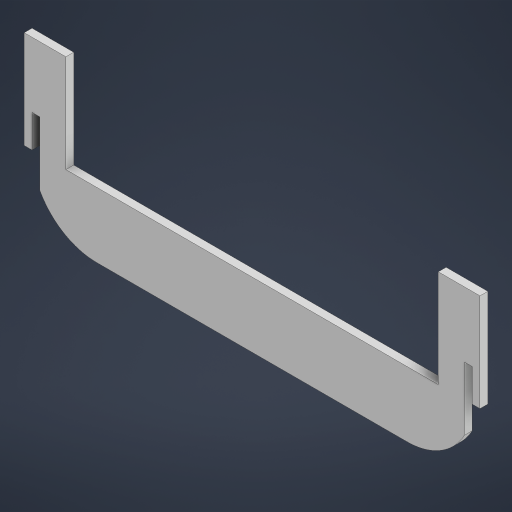
# Autodesk Inventor part: Battery_container_main
Saved by Autodesk Inventor 2024 (Build 280153000, 153)
## iProperties
Created: 2024-02-27
Part Number: Battery_container_main
Material: Generic
Document SubType Name: Modeling
Designer: calvi
Density: 1 g/cm^3
Appearance: Default
Author: calvi
Autodesk Inventor part; units mm, degrees
ref_plane "YZ Plane" through (0, 0, 0) normal (1, 0, 0) x (0, 1, 0)
ref_plane "XZ Plane" through (0, 0, 0) normal (0, 1, 0) x (-1, 0, 0)
ref_plane "XY Plane" through (0, 0, 0) normal (0, 0, 1) x (1, 0, 0)
sketch "Sketch1" plane through (0, 0, 0) normal (0, 0, 1) x (1, 0, 0)
  line L0 (0, 0) -> (171.704, 0)
  line L1 (171.704, 0) -> (171.704, 63.5)
  line L2 (171.704, 63.5) -> (0, 63.5)
  line L3 (0, 63.5) -> (0, 0)
  arc A0 (0, 25.4) -> (25.4, 0) centre (25.4, 25.4) ccw
  arc A1 (146.304, 0) -> (171.704, 25.4) centre (146.304, 25.4) ccw
  dimension "d0" = 171.704
  dimension "d1" = 63.5
  dimension "d2" = 50.8
  dimension "d3" = 50.8
  constraints: 8 end point, 4 point on circle, 4 point on line, 4 tangent, 2 centre point, 2 parallel, 1 horizontal, 1 perpendicular
  measures "d0" distance of L2.end L1.end
  measures "d1" distance of L1.end L0.end
  measures "d2" diameter of A0
  measures "d3" diameter of A1
extrude "Extrusion1" add sketch "Sketch1" along normal blind 3.048 contours A0 L3 L2 L1 A1 L0
sketch "Sketch3" plane through (0, 25.4, 0) normal (-1, 0, 0) x (0, 0, 1)
  line L0 (0, 38.1) -> (0, 0) projected
  line L1 (3.048, -25.4) -> (3.048, 0) projected
  line L2 (0, 38.1) -> (3.048, 38.1)
  line L3 (3.048, 38.1) -> (3.048, 0)
  line L4 (3.048, 0) -> (0, 0)
  line L5 (0, 0) -> (0, 38.1)
  point P0 (0, -25.4)
  constraints: 8 end point, 2 parallel, 1 horizontal, 1 perpendicular
extrude "Extrusion3" add sketch "Sketch3" along normal blind 3.048
sketch "Sketch4" plane through (171.704, 25.4, 0) normal (1, 0, 0) x (0, 0, -1)
  line L0 (-3.048, 38.1) -> (0, 38.1) projected
  line L1 (0, 0) -> (0, -25.4) projected
  line L2 (-3.048, 38.1) -> (0, 38.1)
  line L3 (0, 38.1) -> (0, 0)
  line L4 (0, 0) -> (-3.048, 0)
  line L5 (-3.048, 0) -> (-3.048, 38.1)
  point P0 (0, -25.4)
  constraints: 8 end point, 2 parallel, 1 horizontal, 1 perpendicular
extrude "Extrusion4" add sketch "Sketch4" along normal blind 3.048
sketch "Sketch5" plane through (0, 0, 3.048) normal (0, 0, 1) x (1, 0, 0)
  line L0 (0, 0) -> (3.048, 0)
  line L1 (3.048, 0) -> (3.048, 38.1)
  line L2 (3.048, 38.1) -> (0, 38.1)
  line L3 (0, 38.1) -> (0, 0)
  line L4 (-3.048, 63.5) -> (174.752, 63.5) projected
  line L5 (85.852, 63.5) -> (85.852, 0)
  line L6 (25.4, 0) -> (146.304, 0) projected
  line L7 (171.704, 0) -> (168.656, 0)
  line L8 (168.656, 0) -> (168.656, 38.1)
  line L9 (168.656, 38.1) -> (171.704, 38.1)
  line L10 (171.704, 38.1) -> (171.704, 0)
  point P0 (1.524, 0)
  point P1 (170.18, 0)
  dimension "d17" = 38.1
  dimension "d18" = 3.048
  constraints: 18 end point, 5 symmetric about line, 3 midpoint, 2 parallel, 1 horizontal, 1 perpendicular
  measures "d17" distance from line of L2 point (1.524, 0)
  measures "d18" distance between parallel lines of L3 L1
extrude "Extrusion5" cut sketch "Sketch5" against normal through all
sketch "Sketch6" plane through (0, 0, 3.048) normal (0, 0, 1) x (1, 0, 0)
  line L0 (-3.048, 63.5) -> (174.752, 63.5) projected
  line L1 (13.208, 63.5) -> (158.496, 63.5)
  line L2 (158.496, 63.5) -> (158.496, 25.4)
  line L3 (158.496, 25.4) -> (13.208, 25.4)
  line L4 (13.208, 25.4) -> (13.208, 63.5)
  line L5 (3.048, 38.1) -> (3.048, 13.3357) projected
  line L6 (168.656, 13.3357) -> (168.656, 38.1) projected
  line L7 (25.4, 0) -> (146.304, 0) projected
  point P0 (0, 0)
  point P1 (158.496, 63.5)
  dimension "d21" = 10.16
  dimension "d22" = 10.16
  dimension "d23" = 25.4
  constraints: 8 end point, 2 parallel, 1 horizontal, 1 perpendicular, 1 point on line
  measures "d21" distance between parallel lines of L4 L5
  measures "d22" distance between parallel lines of L6 L2
  measures "d23" distance between parallel lines of L7 L3
extrude "Extrusion6" cut sketch "Sketch6" against normal through all
body "Solid1"
